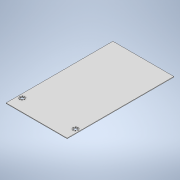
# Autodesk Inventor part: baseplate
Saved by Autodesk Inventor 2020 (Build 240168000, 168)
## iProperties
Created: 2019-09-15
Part Number: baseplate
Material: Generic
Document SubType Name: Modeling
Designer: tdmp4
Density: 1 g/cm^3
Appearance: Default
Author: tdmp4
Autodesk Inventor part; units mm, degrees
ref_plane "YZ Plane" through (0, 0, 0) normal (1, 0, 0) x (0, 1, 0)
ref_plane "XZ Plane" through (0, 0, 0) normal (0, 1, 0) x (-1, 0, 0)
ref_plane "XY Plane" through (0, 0, 0) normal (0, 0, 1) x (1, 0, 0)
sketch "Sketch1" plane through (0, 0, 0) normal (0, 1, 0) x (-1, 0, 0)
  line L0 (-127, 222.25) -> (127, 222.25)
  line L1 (127, 222.25) -> (127, -222.25)
  line L2 (127, -222.25) -> (-127, -222.25)
  line L3 (-127, -222.25) -> (-127, 222.25)
  line L4 (-127, 222.25) -> (127, -222.25) construction
  line L5 (127, 222.25) -> (-127, -222.25) construction
  point P0 (0, 0)
  dimension "d0" = 254
  dimension "d1" = 444.5
  constraints: 12 end point, 2 midpoint, 2 parallel, 1 horizontal, 1 perpendicular
  measures "d0" distance of L1.end L2.end
  measures "d1" distance of L2.end L0.start
extrude "Extrusion1" add sketch "Sketch1" along normal blind 2.286
sketch "Sketch2" plane through (0, 2.286, 0) normal (0, 1, 0) x (1, 0, 0)
  circle A0 centre (-111.0002, -171.555) radius 6.35
  circle A1 centre (111.4204, -171.5462) radius 6.35
  circle A2 centre (-110.9948, -181.3245) radius 1.7859
  circle A3 centre (-110.9948, -161.7665) radius 1.7859
  circle A4 centre (-101.2158, -171.5455) radius 1.7859
  circle A5 centre (-120.7738, -171.5455) radius 1.7859
  circle A6 centre (-117.3448, -164.1087) radius 1.7859
  circle A7 centre (-117.3448, -178.9823) radius 1.7859
  circle A8 centre (-104.6448, -164.1087) radius 1.7859
  circle A9 centre (-104.6448, -178.9823) radius 1.7859
  circle A10 centre (-111.0002, -171.555) radius 6.35
  circle A11 centre (-110.9948, -181.3245) radius 1.7859
  circle A12 centre (-110.9948, -161.7665) radius 1.7859
  circle A13 centre (-101.2158, -171.5455) radius 1.7859
  circle A14 centre (-120.7738, -171.5455) radius 1.7859
  circle A15 centre (-117.3448, -164.1087) radius 1.7859
  circle A16 centre (-117.3448, -178.9823) radius 1.7859
  circle A17 centre (-104.6448, -164.1087) radius 1.7859
  circle A18 centre (-104.6448, -178.9823) radius 1.7859
  circle A19 centre (111.415, -171.5455) radius 6.35
  circle A20 centre (111.4204, -181.315) radius 1.7859
  circle A21 centre (111.4204, -161.757) radius 1.7859
  circle A22 centre (121.1994, -171.536) radius 1.7859
  circle A23 centre (101.6414, -171.536) radius 1.7859
  circle A24 centre (105.0704, -164.0992) radius 1.7859
  circle A25 centre (117.7704, -164.0992) radius 1.7859
  circle A26 centre (117.7704, -178.9728) radius 1.7859
  circle A27 centre (105.0704, -164.0992) radius 1.7859
  circle A28 centre (101.6414, -171.536) radius 1.7859
  circle A29 centre (105.0704, -178.9728) radius 1.7859
  point P0 (0, 0)
  point P1 (112.2628, -165.2523)
  point P2 (110.5726, -177.8394)
  point P3 (-110.9948, -183.1104)
  dimension "d32" = 3.5719
  dimension "d5" = 12.7
  dimension "d6" = 12.7
  dimension "d23" = 3.5719
  dimension "d24" = 3.5719
  dimension "d25" = 3.5719
  dimension "d26" = 3.5719
  dimension "d27" = 3.5719
  dimension "d28" = 3.5719
  dimension "d29" = 3.5719
  dimension "d30" = 3.5719
  dimension "d31" = 12.7
  dimension "d33" = 3.5719
  dimension "d34" = 3.5719
  dimension "d35" = 3.5719
  dimension "d36" = 3.5719
  dimension "d37" = 3.5719
  dimension "d38" = 3.5719
  dimension "d39" = 3.5719
  dimension "d49" = 12.7
  dimension "d50" = 3.5719
  dimension "d51" = 3.5719
  dimension "d52" = 3.5719
  dimension "d53" = 3.5719
  dimension "d54" = 3.5719
  dimension "d56" = 3.5719
  dimension "d57" = 3.5719
  dimension "d62" = 3.5719
  dimension "d63" = 3.5719
  dimension "d64" = 3.5719
  constraints: 29 centre point, 1 vertical alignment, 2 other
  measures "d5" diameter of A0
  measures "d6" diameter of A1
  measures "d23" diameter of A2
  measures "d24" diameter of A3
  measures "d25" diameter of A4
  measures "d26" diameter of A5
  measures "d27" diameter of A6
  measures "d28" diameter of A7
  measures "d29" diameter of A8
  measures "d30" diameter of A9
  measures "d31" diameter of A10
  measures "d33" diameter of A12
  measures "d34" diameter of A13
  measures "d35" diameter of A14
  measures "d36" diameter of A15
  measures "d37" diameter of A16
  measures "d38" diameter of A17
  measures "d39" diameter of A18
  measures "d49" diameter of A19
  measures "d50" diameter of A20
  measures "d51" diameter of A21
  measures "d52" diameter of A22
  measures "d53" diameter of A23
  measures "d54" diameter of A24
  measures "d56" diameter of A25
  measures "d57" diameter of A26
  measures "d62" diameter of A28
  measures "d63" diameter of A27
  measures "d64" diameter of A29
extrude "Extrusion2" cut sketch "Sketch2" against normal blind 2.286
body "Solid1"
